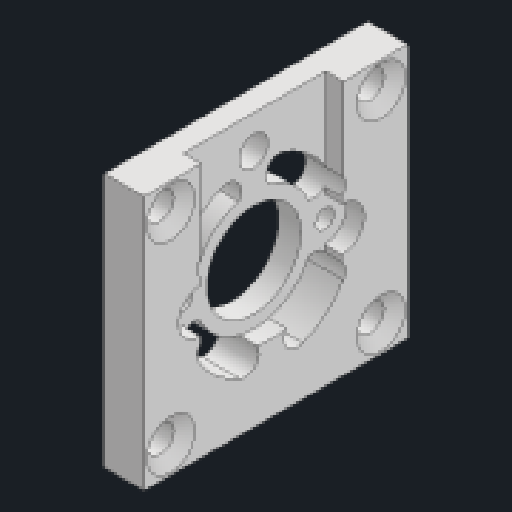
# Autodesk Inventor part: right_motor_mount
Saved by Autodesk Inventor 2023 (Build 270158000, 158)
## iProperties
Created: 2024-04-27
Part Number: right_motor_mount
Material: Generic
Document SubType Name: Modeling
Designer: szymo
Density: 1 g/cm^3
Appearance: Default
Author: szymo
Autodesk Inventor part; units mm, degrees
ref_plane "YZ Plane" through (0, 0, 0) normal (1, 0, 0) x (0, 1, 0)
ref_plane "XZ Plane" through (0, 0, 0) normal (0, 1, 0) x (-1, 0, 0)
ref_plane "XY Plane" through (0, 0, 0) normal (0, 0, 1) x (1, 0, 0)
ref_plane "Work Plane12" through (-37.7, -67.375, 15.375) normal (1, 0, 0) x (0, 0, -1)
sketch "Sketch9" plane through (-37.7, -67.375, 15.375) normal (1, 0, 0) x (0, 0, -1)
  arc A0 (-5.9062, -3.651) -> (-7.7035, -4.7619) centre (-6.8048, -4.2064) ccw projected
  arc A1 (-5.9062, -3.651) -> (-2.5768, -6.4477) centre (0, 0) ccw projected
  arc A2 (-3.3608, -8.4097) -> (-2.5768, -6.4477) centre (-2.9688, -7.4287) ccw projected
  arc A3 (-7.7035, -4.7619) -> (-3.3608, -8.4097) centre (0, 0) ccw projected
  arc A4 (-2.5768, 6.4477) -> (-3.3608, 8.4097) centre (-2.9688, 7.4287) ccw projected
  arc A5 (-2.5768, 6.4477) -> (-5.9062, 3.651) centre (0, 0) ccw projected
  arc A6 (-7.7035, 4.7619) -> (-5.9062, 3.651) centre (-6.8048, 4.2064) ccw projected
  arc A7 (-3.3608, 8.4097) -> (-7.7035, 4.7619) centre (0, 0) ccw projected
  arc A8 (2.5553, -6.4563) -> (3.3328, -8.4209) centre (2.9441, -7.4386) ccw projected
  arc A9 (2.5553, -6.4563) -> (5.9062, -3.651) centre (0, 0) ccw projected
  arc A10 (7.7035, -4.7619) -> (5.9062, -3.651) centre (6.8048, -4.2064) ccw projected
  arc A11 (3.3328, -8.4209) -> (7.7035, -4.7619) centre (0, 0) ccw projected
  arc A12 (5.9062, 3.651) -> (7.7035, 4.7619) centre (6.8048, 4.2064) ccw projected
  arc A13 (5.9062, 3.651) -> (2.5553, 6.4563) centre (0, 0) ccw projected
  arc A14 (3.3328, 8.4209) -> (2.5553, 6.4563) centre (2.9441, 7.4386) ccw projected
  arc A15 (7.7035, 4.7619) -> (3.3328, 8.4209) centre (0, 0) ccw projected
  circle A16 centre (-0.0124, 10.65) radius 1.15 projected
  circle A17 centre (-8, 0) radius 1.0564 projected
  circle A18 centre (8, 0) radius 1.0564 projected
  circle A19 centre (0, 0) radius 5 projected
  circle A20 centre (0, 0) radius 13.7 projected
  line L0 (0, -14.375) -> (15.375, -14.375) projected
  line L1 (15.375, -14.375) -> (15.375, 14.375) projected
  line L2 (15.375, 14.375) -> (0, 14.375) projected
  line L3 (0, 14.375) -> (0, 13.7) projected
  arc A21 (0, -13.7) -> (0, 13.7) centre (0, 0) ccw projected
  line L4 (0, -13.7) -> (0, -14.375) projected
  line L5 (18.375, -91.625) -> (18.375, 14.375) projected
  line L6 (18.375, 14.375) -> (15.375, 14.375) projected
  line L7 (15.375, -91.625) -> (15.375, 14.375) projected
  line L8 (18.375, -91.625) -> (15.375, -91.625) projected
  arc A22 (0.512, -3.83) -> (1.6707, -5.5993) centre (4.9979, -2.1562) ccw projected
  arc A23 (1.6707, -5.5993) -> (2.5261, -5.269) centre (0, 0) ccw projected
  arc A24 (2.5261, -5.269) -> (2.195, -3.1802) centre (-2.2517, -4.9556) ccw projected
  arc A25 (2.195, -3.1802) -> (2.6654, -2.7976) centre (0, 0) ccw projected
  arc A26 (2.6654, -2.7976) -> (4.6428, -3.548) centre (5.3108, 1.1933) ccw projected
  arc A27 (4.6428, -3.548) -> (5.1407, -2.778) centre (0, 0) ccw projected
  arc A28 (5.1407, -2.778) -> (3.645, -1.2826) centre (1.0912, -5.3327) ccw projected
  arc A29 (3.645, -1.2826) -> (3.8008, -0.6966) centre (0, 0) ccw projected
  arc A30 (3.8008, -0.6966) -> (5.8416, -0.1414) centre (3.5951, 4.087) ccw projected
  arc A31 (5.8416, -0.1414) -> (5.7918, 0.7742) centre (0, 0) ccw projected
  arc A32 (5.7918, 0.7742) -> (3.7028, 1.1048) centre (4.0173, -3.6729) ccw projected
  arc A33 (3.7028, 1.1048) -> (3.4844, 1.6705) centre (0, 0) ccw projected
  arc A34 (3.4844, 1.6705) -> (4.809, 3.3192) centre (0.5063, 5.4196) ccw projected
  arc A35 (4.809, 3.3192) -> (4.2306, 4.0306) centre (0, 0) ccw projected
  arc A36 (4.2306, 4.0306) -> (2.3462, 3.0703) centre (5.4089, -0.6101) ccw projected
  arc A37 (2.3462, 3.0703) -> (1.8371, 3.3995) centre (0, 0) ccw projected
  arc A38 (1.8371, 3.3995) -> (1.9396, 5.512) centre (-2.776, 4.6821) ccw projected
  arc A39 (1.9396, 5.512) -> (1.0535, 5.7475) centre (0, 0) ccw projected
  arc A40 (1.0535, 5.7475) -> (0.0935, 3.863) centre (4.7345, 2.6857) ccw projected
  arc A41 (0.0935, 3.863) -> (-0.512, 3.83) centre (0, 0) ccw projected
  arc A42 (-0.512, 3.83) -> (-1.6707, 5.5993) centre (-4.9979, 2.1562) ccw projected
  arc A43 (-1.6707, 5.5993) -> (-2.5261, 5.269) centre (0, 0) ccw projected
  arc A44 (-2.5261, 5.269) -> (-2.195, 3.1802) centre (2.2517, 4.9556) ccw projected
  arc A45 (-2.195, 3.1802) -> (-2.6654, 2.7976) centre (0, 0) ccw projected
  arc A46 (-2.6654, 2.7976) -> (-4.6428, 3.548) centre (-5.3108, -1.1933) ccw projected
  arc A47 (-4.6428, 3.548) -> (-5.1407, 2.778) centre (0, 0) ccw projected
  arc A48 (-5.1407, 2.778) -> (-3.645, 1.2826) centre (-1.0912, 5.3327) ccw projected
  arc A49 (-3.645, 1.2826) -> (-3.8008, 0.6966) centre (0, 0) ccw projected
  arc A50 (-3.8008, 0.6966) -> (-5.8416, 0.1414) centre (-3.5951, -4.087) ccw projected
  arc A51 (-5.8416, 0.1414) -> (-5.7918, -0.7742) centre (0, 0) ccw projected
  arc A52 (-5.7918, -0.7742) -> (-3.7028, -1.1048) centre (-4.0173, 3.6729) ccw projected
  arc A53 (-3.7028, -1.1048) -> (-3.4844, -1.6705) centre (0, 0) ccw projected
  arc A54 (-3.4844, -1.6705) -> (-4.809, -3.3192) centre (-0.5063, -5.4196) ccw projected
  arc A55 (-4.809, -3.3192) -> (-4.2306, -4.0306) centre (0, 0) ccw projected
  arc A56 (-4.2306, -4.0306) -> (-2.3462, -3.0703) centre (-5.4089, 0.6101) ccw projected
  arc A57 (-2.3462, -3.0703) -> (-1.8371, -3.3995) centre (0, 0) ccw projected
  arc A58 (-1.8371, -3.3995) -> (-1.9396, -5.512) centre (2.776, -4.6821) ccw projected
  arc A59 (-1.9396, -5.512) -> (-1.0535, -5.7475) centre (0, 0) ccw projected
  arc A60 (-1.0535, -5.7475) -> (-0.0935, -3.863) centre (-4.7345, -2.6857) ccw projected
  arc A61 (-0.0935, -3.863) -> (0.512, -3.83) centre (0, 0) ccw projected
  circle A62 centre (0, 0) radius 14.375 projected
  line L9 (15.375, -14.375) -> (9.875, -14.375) projected
  line L10 (15.375, -14.375) -> (-14.375, -14.375)
  line L11 (-14.375, -14.375) -> (-14.375, 14.375)
  line L12 (-14.375, 14.375) -> (15.375, 14.375)
  line L13 (15.375, 14.375) -> (15.375, -14.375)
  arc A63 (-3.5464, -8.874) -> (-2.3912, -5.9835) centre (-2.9688, -7.4287) ccw
  arc A64 (-5.4809, -3.3881) -> (-2.3912, -5.9835) centre (0, 0) ccw
  arc A65 (-5.4809, -3.3881) -> (-8.1288, -5.0248) centre (-6.8048, -4.2064) ccw
  arc A66 (-8.1288, -5.0248) -> (-3.5464, -8.874) centre (0, 0) ccw
  arc A67 (-8.1288, 5.0248) -> (-5.4809, 3.3881) centre (-6.8048, 4.2064) ccw
  arc A68 (-2.3912, 5.9835) -> (-5.4809, 3.3881) centre (0, 0) ccw
  arc A69 (-2.3912, 5.9835) -> (-3.5464, 8.874) centre (-2.9688, 7.4287) ccw
  arc A70 (-3.5464, 8.874) -> (-8.1288, 5.0248) centre (0, 0) ccw
  arc A71 (2.3713, -5.9914) -> (5.4809, -3.3881) centre (0, 0) ccw
  arc A72 (2.3713, -5.9914) -> (3.5168, -8.8858) centre (2.9441, -7.4386) ccw
  arc A73 (3.5168, -8.8858) -> (8.1288, -5.0248) centre (0, 0) ccw
  arc A74 (8.1288, -5.0248) -> (5.4809, -3.3881) centre (6.8048, -4.2064) ccw
  arc A75 (3.5168, 8.8858) -> (2.3713, 5.9914) centre (2.9441, 7.4386) ccw
  arc A76 (5.4809, 3.3881) -> (2.3713, 5.9914) centre (0, 0) ccw
  arc A77 (5.4809, 3.3881) -> (8.1288, 5.0248) centre (6.8048, 4.2064) ccw
  arc A78 (8.1288, 5.0248) -> (3.5168, 8.8858) centre (0, 0) ccw
  circle A79 centre (-0.0124, 10.65) radius 1.65
  circle A80 centre (0, 0) radius 6.75 projected
  circle A81 centre (0, 0) radius 5.3
  point P0 (15.375, 67.375)
  point P1 (0, -14.375)
  point P2 (0, 14.375)
  point P3 (-6.1429, -2.7978)
  point P4 (-1.6956, -6.5336)
  point P5 (6.1429, -2.7978)
  point P6 (1.6738, -6.5392)
  point P7 (1.6738, 6.5392)
  point P8 (6.1429, 2.7978)
  point P9 (-6.1429, 2.7978)
  point P10 (-1.6956, 6.5336)
  dimension "d28" = 0.5
  dimension "d29" = 0.5
  dimension "d30" = 0.5
  dimension "d31" = 0.5
  dimension "d32" = 0.5
  dimension "d33" = 0.3
  constraints: 32 point on circle, 18 centre point, 8 end point, 2 parallel, 2 tangent, 1 horizontal, 1 perpendicular, 12 other
  measures "d28" radial gap between concentric circles of A3 A66
  measures "d29" radial gap between concentric circles of A7 A70
  measures "d30" radial gap between concentric circles of A9 A71
  measures "d31" radial gap between concentric circles of A15 A78
  measures "d32" radial gap between concentric circles of A16 A79
  measures "d33" radial gap between concentric circles of A19 A81
extrude "Extrusion6" add sketch "Sketch9" along normal blind 2.5 contours A32 A31 A30 A81 | A81 A36 A35 A34 | A28 A27 A26 A81 | A81 A40 A39 A38 | A24 A23 A22 A81 | A81 A44 A43 A42 | A60 A59 A58 A81 | A81 A48 A47 A46 | A56 A55 A54 A81 | A81 A52 A51 A50 | A20 | A20 L3 A62 L4 | A20 L4 A62 L3 | L2 L1 L0 A62 | A62 L11 L12 | L10 L11 A62 | A80 A65 A64 A63 | A63 A64 A65 A80 A67 A68 A69 A75 A76 A77 A74 A71 A72 | A72 A71 A74 A80 | A80 A69 A68 A67 | A80 A77 A76 A75
ref_plane "Work Plane13" through (-35.2, -67.375, 15.375) normal (1, 0, 0) x (0, 0, -1)
sketch "Sketch10" plane through (-35.2, -67.375, 15.375) normal (1, 0, 0) x (0, 0, -1)
  line L0 (15.375, -14.375) -> (15.375, 14.375) projected
  line L1 (15.375, 14.375) -> (-14.375, 14.375) projected
  line L2 (-14.375, 14.375) -> (-14.375, -14.375) projected
  line L3 (-14.375, -14.375) -> (15.375, -14.375) projected
  circle A0 centre (-8, 0) radius 1.0564 projected
  circle A1 centre (8, 0) radius 1.0564 projected
  circle A2 centre (-0.0124, 10.65) radius 1.65 projected
  arc A3 (-6.1429, -2.7978) -> (-1.6956, -6.5336) centre (0, 0) ccw projected
  arc A4 (-3.5464, -8.874) -> (-1.6956, -6.5336) centre (-2.9688, -7.4287) ccw projected
  arc A5 (-8.1288, -5.0248) -> (-3.5464, -8.874) centre (0, 0) ccw projected
  arc A6 (-6.1429, -2.7978) -> (-8.1288, -5.0248) centre (-6.8048, -4.2064) ccw projected
  circle A7 centre (0, 0) radius 5.3 projected
  arc A8 (8.1288, -5.0248) -> (6.1429, -2.7978) centre (6.8048, -4.2064) ccw projected
  arc A9 (3.5168, -8.8858) -> (8.1288, -5.0248) centre (0, 0) ccw projected
  arc A10 (1.6738, -6.5392) -> (3.5168, -8.8858) centre (2.9441, -7.4386) ccw projected
  arc A11 (1.6738, -6.5392) -> (6.1429, -2.7978) centre (0, 0) ccw projected
  arc A12 (3.5168, 8.8858) -> (1.6738, 6.5392) centre (2.9441, 7.4386) ccw projected
  arc A13 (8.1288, 5.0248) -> (3.5168, 8.8858) centre (0, 0) ccw projected
  arc A14 (6.1429, 2.7978) -> (8.1288, 5.0248) centre (6.8048, 4.2064) ccw projected
  arc A15 (6.1429, 2.7978) -> (1.6738, 6.5392) centre (0, 0) ccw projected
  arc A16 (-8.1288, 5.0248) -> (-6.1429, 2.7978) centre (-6.8048, 4.2064) ccw projected
  arc A17 (-3.5464, 8.874) -> (-8.1288, 5.0248) centre (0, 0) ccw projected
  arc A18 (-1.6956, 6.5336) -> (-3.5464, 8.874) centre (-2.9688, 7.4287) ccw projected
  arc A19 (-1.6956, 6.5336) -> (-6.1429, 2.7978) centre (0, 0) ccw projected
  circle A20 centre (0, 0) radius 6.75 projected
  circle A21 centre (-8, 0) radius 1.0564 projected
  circle A22 centre (-8, 0) radius 2.5
  circle A23 centre (8, 0) radius 1.0564 projected
  circle A24 centre (8, 0) radius 2.5
  arc A25 (-6.1429, -2.7978) -> (-8.1288, -5.0248) centre (-6.8048, -4.2064) ccw projected
  line L4 (-7.9665, -3.1706) -> (-7.9665, -2.4998)
  arc A26 (-8.1288, 5.0248) -> (-6.1429, 2.7978) centre (-6.8048, 4.2064) ccw projected
  line L5 (-7.9665, 3.1706) -> (-7.9665, 2.4998)
  arc A27 (6.1429, 2.7978) -> (8.1288, 5.0248) centre (6.8048, 4.2064) ccw projected
  line L6 (7.9665, 3.1706) -> (7.9665, 2.4998)
  line L7 (7.9665, -3.1706) -> (7.9665, -2.4998)
  line L8 (8.1288, 5.0248) -> (8.1288, 14.375)
  line L9 (0, 14.375) -> (15.375, 14.375) projected
  line L10 (-7.9665, 5.2783) -> (-7.9665, 14.375)
  line L11 (0, 14.375) -> (-14.375, 14.375) projected
  point P0 (15.375, 67.375)
  point P1 (-6.457, -1.967)
  point P2 (-6.457, 1.967)
  point P3 (6.457, 1.967)
  point P4 (6.457, -1.967)
  point P5 (8.1288, 14.375)
  point P6 (-7.9665, 14.375)
  dimension "d36" = 5
  dimension "d37" = 5
  constraints: 12 end point, 12 point on circle, 3 point on line, 2 centre point, 2 coincident, 2 perpendicular, 2 vertical, 1 parallel, 1 other
  measures "d36" diameter of A22
  measures "d37" diameter of A24
extrude "Extrusion7" add sketch "Sketch10" along normal blind 2 contours L3 L2 L1 L10 A17 A16 L5 A22 L4 A6 A5 A4 A20 A10 A9 A8 L7 A24 L6 A14 L8 L0
sketch "Sketch15" plane through (-33.2, -67.375, 15.375) normal (1, 0, 0) x (0, 0, -1)
  line L0 (15.375, 14.375) -> (8.1288, 14.375) projected
  line L1 (8.1288, 14.375) -> (8.1288, 5.0248) projected
  arc A0 (7.9665, 3.1706) -> (8.1288, 5.0248) centre (6.8048, 4.2064) ccw projected
  line L2 (7.9665, 3.1706) -> (7.9665, 2.4998) projected
  arc A1 (7.9665, -2.4998) -> (7.9665, 2.4998) centre (8, 0) ccw projected
  line L3 (7.9665, -2.4998) -> (7.9665, -3.1706) projected
  arc A2 (8.1288, -5.0248) -> (7.9665, -3.1706) centre (6.8048, -4.2064) ccw projected
  arc A3 (3.5168, -8.8858) -> (8.1288, -5.0248) centre (0, 0) ccw projected
  arc A4 (1.6738, -6.5392) -> (3.5168, -8.8858) centre (2.9441, -7.4386) ccw projected
  arc A5 (-1.6956, -6.5336) -> (1.6738, -6.5392) centre (0, 0) ccw projected
  arc A6 (-3.5464, -8.874) -> (-1.6956, -6.5336) centre (-2.9688, -7.4287) ccw projected
  arc A7 (-8.1288, -5.0248) -> (-3.5464, -8.874) centre (0, 0) ccw projected
  arc A8 (-7.9665, -3.1706) -> (-8.1288, -5.0248) centre (-6.8048, -4.2064) ccw projected
  line L4 (-7.9665, -3.1706) -> (-7.9665, -2.4998) projected
  arc A9 (-7.9665, 2.4998) -> (-7.9665, -2.4998) centre (-8, 0) ccw projected
  line L5 (-7.9665, 2.4998) -> (-7.9665, 3.1706) projected
  arc A10 (-8.1288, 5.0248) -> (-7.9665, 3.1706) centre (-6.8048, 4.2064) ccw projected
  arc A11 (-7.9665, 5.2783) -> (-8.1288, 5.0248) centre (0, 0) ccw projected
  line L6 (-7.9665, 5.2783) -> (-7.9665, 14.375) projected
  line L7 (-7.9665, 14.375) -> (-14.375, 14.375) projected
  line L8 (-14.375, 14.375) -> (-14.375, -14.375) projected
  line L9 (-14.375, -14.375) -> (15.375, -14.375) projected
  line L10 (15.375, -14.375) -> (15.375, 14.375) projected
  circle A12 centre (-11.375, 11.375) radius 3
  circle A13 centre (-11.375, -11.375) radius 3
  circle A14 centre (12.375, -11.375) radius 3
  circle A15 centre (12.375, 11.375) radius 3
  point P0 (15.375, 67.375)
  dimension "d58" = 6
  dimension "d59" = 6
  dimension "d60" = 6
  dimension "d61" = 6
  dimension "d62" = 3
  dimension "d63" = 3
  dimension "d64" = 3
  dimension "d65" = 3
  dimension "d66" = 3
  dimension "d67" = 3
  dimension "d68" = 3
  dimension "d69" = 3
  constraints: 4 centre point
  measures "d58" diameter of A12
  measures "d59" diameter of A13
  measures "d60" diameter of A14
  measures "d61" diameter of A15
  measures "d62" distance from line of L8 A13.centre
  measures "d63" distance from line of L9 A13.centre
  measures "d64" distance from line of L8 A12.centre
  measures "d65" distance from line of L7 A12.centre
  measures "d66" distance from line of L10 A14.centre
  measures "d67" distance from line of L9 A14.centre
  measures "d68" distance from line of L0 A15.centre
  measures "d69" distance from line of L10 A15.centre
hole "Hole4" at (-33.2, -78.75, 26.75) at (-33.2, -78.75, 3) at (-33.2, -56, 3) at (-33.2, -56, 26.75) direction (-1, 0, 0) diameter 3.1 end through all countersink diameter 5.5 countersink angle 90 clearance for "Countersunk Flat Head Screw ISO 2009/7046" size "M2.5" standard "ISO"
equation "\"d62\" = 0.5 * d59"
equation "\"d63\" = 0.5 * d59"
equation "\"d64\" = 0.5 * d58"
equation "\"d65\" = 0.5 * d58"
equation "\"d66\" = 0.5 * d60"
equation "\"d67\" = 0.5 * d60"
equation "\"d68\" = 0.5 * d61"
equation "\"d69\" = 0.5 * d61"
body "Solid1"
